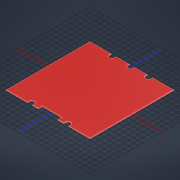
# Autodesk Inventor part: Silicon-Heater (350mm)
Saved by Autodesk Inventor 2022.2 (Build 262287010, 287A)
## iProperties
Created: 2022-03-13
Part Number: Silicon-Heater (350mm)
Material: Gummi, Silikon
Document SubType Name: Modeling
Designer: sleib
Density: 1.25 g/cm^3
Appearance: Orangerot
Author: sleib
Autodesk Inventor part; units mm, degrees
ref_plane "YZ Plane" through (0, 0, 0) normal (1, 0, 0) x (0, 1, 0)
ref_plane "XZ Plane" through (0, 0, 0) normal (0, 1, 0) x (-1, 0, 0)
ref_plane "XY Plane" through (0, 0, 0) normal (0, 0, 1) x (1, 0, 0)
sketch "Skizze1" plane through (0, 0, 0) normal (0, 1, 0) x (-1, 0, 0)
  line L0 (174.5, 174.5) -> (-174.5, 174.5)
  line L1 (-174.5, 174.5) -> (-174.5, -174.5)
  line L2 (-174.5, -174.5) -> (174.5, -174.5)
  line L3 (174.5, -174.5) -> (174.5, 174.5)
  line L4 (174.5, 174.5) -> (-174.5, -174.5) construction
  line L5 (-174.5, 174.5) -> (174.5, -174.5) construction
  line L6 (244.3, 0) -> (-244.3, 0) construction
  line L7 (0, -244.3) -> (0, 244.3) construction
  arc A0 (10, -167) -> (-10, -167) centre (0, -167) ccw
  arc A1 (85, -167) -> (65, -167) centre (75, -167) ccw
  arc A2 (-65, -167) -> (-85, -167) centre (-75, -167) ccw
  line L8 (85, -167) -> (85, -174.5)
  line L9 (65, -167) -> (65, -174.5)
  line L10 (10, -167) -> (10, -174.5)
  line L11 (-10, -167) -> (-10, -174.5)
  line L12 (-65, -167) -> (-65, -174.5)
  line L13 (-85, -167) -> (-85, -174.5)
  line L14 (-65, -174.5) -> (-85, -174.5)
  line L15 (10, -174.5) -> (-10, -174.5)
  line L16 (85, -174.5) -> (65, -174.5)
  line L17 (40, 174.5) -> (-40, 174.5)
  line L18 (-40, 174.5) -> (-40, 157.5)
  line L19 (-40, 157.5) -> (40, 157.5)
  line L20 (40, 157.5) -> (40, 174.5)
  arc A3 (65, 167) -> (85, 167) centre (75, 167) ccw
  arc A4 (-85, 167) -> (-65, 167) centre (-75, 167) ccw
  line L21 (85, 167) -> (85, 174.5)
  line L22 (65, 167) -> (65, 174.5)
  line L23 (-65, 167) -> (-65, 174.5)
  line L24 (-85, 167) -> (-85, 174.5)
  line L25 (-65, 174.5) -> (-85, 174.5)
  line L26 (85, 174.5) -> (65, 174.5)
  point P0 (0, 0)
  dimension "d0" = 349
  dimension "d1" = 349
  dimension "d2" = 20
  dimension "d3" = 17.5
  dimension "d4" = 150
  dimension "d5" = 17
  dimension "d6" = 80
  constraints: 50 end point, 11 symmetric about line, 10 point on circle, 9 perpendicular, 8 point on line, 6 tangent, 5 centre point, 4 parallel, 2 collinear, 2 equal radius, 2 horizontal, 2 horizontal alignment, 2 midpoint, 3 other
  measures "d0" distance of L2.end L1.end
  measures "d1" distance of L1.end L0.end
  measures "d2" diameter of A0
  measures "d4" distance of A2.centre A1.centre
  measures "d5" distance between parallel lines of L0 L19
  measures "d6" distance between parallel lines of L18 L20
extrude "Extrusion1" add sketch "Skizze1" along normal blind 2 contours L3 L2 L8 A1 L9 L10 A0 L11 L12 A2 L13 L1 L0 L24 A4 L23 L18 L19 L20 L22 A3 L21
fillet "Rundung1" radius 1.5 28 edges at (-129.75, 2, 174.5) (-75, 2, 157) (-65, 2, 170.75) (-85, 2, 170.75) (-52.5, 2, 174.5) (-40, 2, 166) (0, 2, 157.5) (40, 2, 166) (52.5, 2, 174.5) (75, 2, 157) (85, 2, 170.75) (65, 2, 170.75) (129.75, 2, 174.5) (174.5, 2, 0) (129.75, 2, -174.5) (65, 2, -170.75) (85, 2, -170.75) (75, 2, -157) (37.5, 2, -174.5) (-10, 2, -170.75) (10, 2, -170.75) (0, 2, -157) (-37.5, 2, -174.5) (-85, 2, -170.75) (-65, 2, -170.75) (-75, 2, -157) (-129.75, 2, -174.5) (-174.5, 2, 0)
